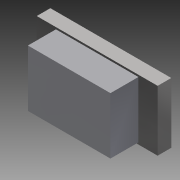
# Autodesk Inventor part: sLarge LED
Saved by Autodesk Inventor 2015 (Build 190159000, 159)
## iProperties
Created: 2016-01-19
Part Number: sLarge LED
Material: Generic
Document SubType Name: Modeling
Designer: Kyle
Density: 1 g/cm^3
Appearance: Default
Author: Kyle
Autodesk Inventor part; units mm, degrees
ref_plane "YZ Plane" through (0, 0, 0) normal (1, 0, 0) x (0, 1, 0)
ref_plane "XZ Plane" through (0, 0, 0) normal (0, 1, 0) x (-1, 0, 0)
ref_plane "XY Plane" through (0, 0, 0) normal (0, 0, 1) x (1, 0, 0)
sketch "Sketch1" plane through (0, 0, 0) normal (0, 0, 1) x (1, 0, 0)
  line L0 (0, 0) -> (1.6002, 0)
  line L1 (1.6002, 0) -> (1.6002, 0.8001)
  line L2 (1.6002, 0.8001) -> (0, 0.8001)
  line L3 (0, 0.8001) -> (0, 0)
  dimension "d0" = 1.6002
  dimension "d1" = 0.8001
  constraints: 8 end point, 2 parallel, 1 horizontal, 1 perpendicular
  measures "d0" distance of L1.end L2.end
  measures "d1" distance of L0.end L1.end
extrude "Extrusion1" add sketch "Sketch1" along normal blind 0.1803
sketch "Sketch2" plane through (0, 0, 0.1803) normal (0, 0, 1) x (1, 0, 0)
  line L0 (0.254, 0.7747) -> (1.3462, 0.7747)
  line L1 (1.3462, 0.7747) -> (1.3462, 0.0254)
  line L2 (1.3462, 0.0254) -> (0.254, 0.0254)
  line L3 (0.254, 0.0254) -> (0.254, 0.7747)
  line L4 (1.6002, 0.8001) -> (0, 0.8001) projected
  line L5 (0, 0) -> (1.6002, 0) projected
  line L6 (1.6002, 0) -> (1.6002, 0.8001) projected
  line L7 (0, 0.8001) -> (0, 0) projected
  dimension "d4" = 0.0254
  dimension "d5" = 0.0254
  dimension "d6" = 0.254
  dimension "d7" = 0.254
  constraints: 8 end point, 2 parallel, 1 horizontal, 1 perpendicular
  measures "d4" distance between parallel lines of L4 L0
  measures "d5" distance between parallel lines of L5 L2
  measures "d6" distance between parallel lines of L6 L1
  measures "d7" distance between parallel lines of L7 L3
extrude "Extrusion2" add sketch "Sketch2" along normal blind 0.3708 contours L0 L1 L2 L3
sketch "Sketch3" plane through (0, 0, 0.1803) normal (0, 0, 1) x (1, 0, 0)
  circle A0 centre (0.127, 0.127) radius 0.0635
  line L0 (0, 0) -> (1.6002, 0) projected
  line L1 (0, 0.8001) -> (0, 0) projected
  dimension "d10" = 0.127
  dimension "d11" = 0.127
  dimension "d12" = 0.127
  constraints: 1 centre point
  measures "d10" diameter of A0
  measures "d11" distance from line of L0 A0.centre
  measures "d12" distance from line of L1 A0.centre
extrude "Extrusion3" cut sketch "Sketch3" against normal blind 0.0254
body "Solid1"
